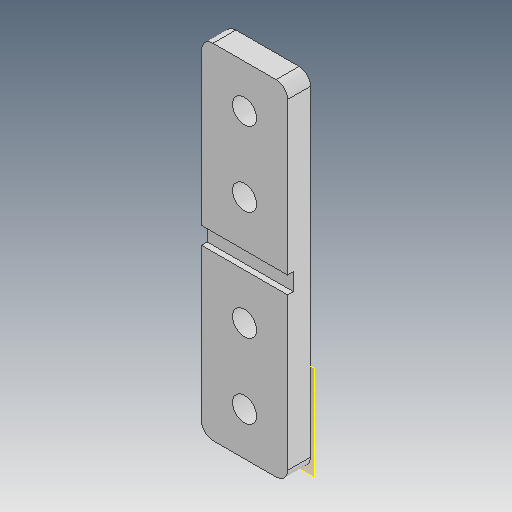
# Autodesk Inventor part: suporte_termopar_al
Saved by Autodesk Inventor 2020 (Build 240168000, 168)
## iProperties
Created: 2022-07-21
Part Number: suporte_termopar_al
Material: Genérico
Document SubType Name: Modeling
Designer: gabri
Density: 1 g/cm^3
Appearance: Padrão
Author: gabri
Autodesk Inventor part; units mm, degrees
ref_plane "YZ Plane" through (0, 0, 0) normal (1, 0, 0) x (0, 1, 0)
ref_plane "XZ Plane" through (0, 0, 0) normal (0, 1, 0) x (-1, 0, 0)
ref_plane "XY Plane" through (0, 0, 0) normal (0, 0, 1) x (1, 0, 0)
ref_plane "Plano de trabalho1" through (0, -45, 0) normal (0, 0, 1) x (1, 0, 0)
sketch "Esboço1" plane through (0, -45, 0) normal (0, 0, 1) x (1, 0, 0)
  arc A0 (5.5, 37.5) -> (7.5, 39.5) centre (5.5, 39.5) ccw projected
  line L0 (7.5, 39.5) -> (7.5, 50.5) projected
  arc A1 (7.5, 50.5) -> (5.5, 52.5) centre (5.5, 50.5) ccw projected
  line L1 (5.5, 52.5) -> (-5.5, 52.5) projected
  arc A2 (-5.5, 52.5) -> (-7.5, 50.5) centre (-5.5, 50.5) ccw projected
  line L2 (-7.5, 50.5) -> (-7.5, 39.5) projected
  arc A3 (-7.5, 39.5) -> (-5.5, 37.5) centre (-5.5, 39.5) ccw projected
  line L3 (-5.5, 37.5) -> (5.5, 37.5) projected
  circle A4 centre (0, 45) radius 2.1 projected
  arc A5 (-7.5, -5.5) -> (-5.5, -7.5) centre (-5.5, -5.5) ccw projected
  line L4 (-5.5, -7.5) -> (5.5, -7.5) projected
  arc A6 (5.5, -7.5) -> (7.5, -5.5) centre (5.5, -5.5) ccw projected
  line L5 (7.5, -5.5) -> (7.5, 5.5) projected
  arc A7 (7.5, 5.5) -> (5.5, 7.5) centre (5.5, 5.5) ccw projected
  line L6 (5.5, 7.5) -> (-5.5, 7.5) projected
  arc A8 (-5.5, 7.5) -> (-7.5, 5.5) centre (-5.5, 5.5) ccw projected
  line L7 (-7.5, 5.5) -> (-7.5, -5.5) projected
  circle A9 centre (0, 0) radius 2.1 projected
  line L8 (7.5, 39.5) -> (7.5, 5.5)
  line L9 (-7.5, 39.5) -> (-7.5, 5.5)
  constraints: 4 end point, 1 collinear, 1 parallel
extrude "Extrusão1" add sketch "Esboço1" along normal blind 4
sketch "Esboço2" plane through (0, -45, 4) normal (0, 0, 1) x (1, 0, 0)
  line L0 (7.5, -5.5) -> (7.5, 50.5) projected
  line L1 (-7.5, 50.5) -> (-7.5, -5.5) projected
  line L2 (7.5, 24) -> (-7.5, 24)
  line L3 (-7.5, 24) -> (-7.5, 21)
  line L4 (-7.5, 21) -> (7.5, 21)
  line L5 (7.5, 21) -> (7.5, 24)
  line L6 (5.5, 52.5) -> (-5.5, 52.5) projected
  line L7 (-5.5, -7.5) -> (5.5, -7.5) projected
  circle A0 centre (0, 32) radius 2.1
  circle A1 centre (0, 13) radius 2.1
  point P0 (0, 45)
  point P1 (7.5, 21)
  dimension "d4" = 28.5
  dimension "d5" = 28.5
  dimension "d6" = 3
  dimension "d7" = 4.2
  dimension "d8" = 4.2
  dimension "d9" = 8
  dimension "d10" = 8
  constraints: 8 end point, 2 centre point, 2 parallel, 2 point on line, 1 horizontal, 1 perpendicular
  measures "d4" distance between parallel lines of L6 L2
  measures "d5" distance between parallel lines of L7 L4
  measures "d6" distance between parallel lines of L4 L2
  measures "d7" diameter of A0
  measures "d8" diameter of A1
  measures "d9" distance from line of L2 A0.centre
  measures "d10" distance from line of L4 A1.centre
extrude "Extrusão2" cut sketch "Esboço2" against normal blind 1
sketch "Esboço3" plane through (0, -13, 3) normal (0, 0, 1) x (1, 0, 0)
  circle A0 centre (0, 0) radius 2.1 projected
  circle A1 centre (0, -19) radius 2.1 projected
  point P0 (0, 13)
extrude "Extrusão3" cut sketch "Esboço3" against normal blind 10
equation "\"d5\" = d4"
equation "\"d10\" = d9"
